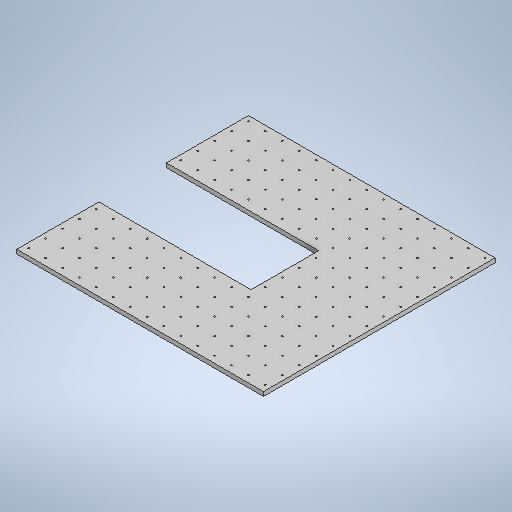
# Autodesk Inventor part: box tray_middle
Saved by Autodesk Inventor 2025.3 (Build 293356000, 356)
## iProperties
Created: 2026-02-03
Part Number: box tray_middle
Material: Generic
Document SubType Name: Modeling
Designer: AdminForWorker
Density: 1 g/cm^3
Appearance: Default
Title: box tray v1
Author: AdminForWorker
Autodesk Inventor part; units mm, degrees
ref_plane "YZ Plane" through (0, 0, 0) normal (1, 0, 0) x (0, 1, 0)
ref_plane "XZ Plane" through (0, 0, 0) normal (0, 1, 0) x (-1, 0, 0)
ref_plane "XY Plane" through (0, 0, 0) normal (0, 0, 1) x (1, 0, 0)
sketch "Sketch2" plane through (0, 0, 0) normal (0, 1, 0) x (-1, 0, 0)
  line L0 (-476, -174) -> (-476, 174) projected
  line L1 (-924, -174) -> (-476, -174) projected
  line L2 (-924, 174) -> (-924, -174) projected
  line L3 (-476, 174) -> (-924, 174) projected
  point P0 (0, 0)
extrude "Extrusion1" add sketch "Sketch2" along normal blind 6.35
sketch "Sketch3" plane through (0, 6.35, 0) normal (0, 1, 0) x (1, 0, 0)
  circle A0 centre (483.62, 166.38) radius 1.1355
  line L0 (924, 174) -> (476, 174) projected
  line L1 (476, 174) -> (476, -174) projected
  point P0 (0, 0)
  dimension "d8" = 2.271
  dimension "d9" = 7.62
  dimension "d10" = 7.62
  constraints: 1 centre point
  measures "d8" diameter of A0
  measures "d9" distance from line of L0 A0.centre
  measures "d10" distance from line of L1 A0.centre
extrude "Extrusion2" cut sketch "Sketch3" against normal blind 6.35
pattern_linear "Rectangular Pattern1" count 14 spacing 25.4 along (0, 0, 1) count 18 spacing 25.4 along (1, 0, 0) of "Extrusion2"
sketch "Sketch6" plane through (0, 6.35, 0) normal (0, 1, 0) x (1, 0, 0)
  line L0 (476, 174) -> (476, -174) projected
  line L1 (476, 50.8) -> (704.6, 50.8)
  line L2 (704.6, 50.8) -> (704.6, -50.8)
  line L3 (704.6, -50.8) -> (476, -50.8)
  line L4 (476, -50.8) -> (476, 50.8)
  circle A0 centre (485, 0) radius 2.138 projected
  line L5 (924, 174) -> (476, 174) projected
  line L6 (924, 174) -> (846.53, 174)
  line L7 (846.53, 174) -> (846.53, -174)
  line L8 (846.53, -174) -> (924, -174)
  line L9 (924, -174) -> (924, 174)
  point P0 (0, 0)
  point P1 (846.53, 174)
  dimension "d25" = 228.6
  dimension "d26" = 101.6
  dimension "d27" = 50.8
  dimension "d29" = 348
  dimension "d32" = 77.47
  constraints: 16 end point, 4 parallel, 2 horizontal, 2 perpendicular, 1 point on line
  measures "d25" distance of L2.end L3.end
  measures "d26" distance of L1.end L2.end
  measures "d27" distance from line of A0.centre L1
  measures "d29" distance of L7.end L6.end
  measures "d32" distance of L7.end L8.end
extrude "Extrusion6" cut sketch "Sketch6" against normal blind 6.35 contours L1 L2 L3 L0 | L5 L9 L8 L7 | A0
body "Solid2"
